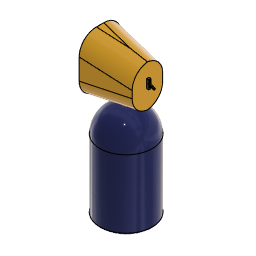
WeirdLamp v2 (Autodesk Fusion 360 design; units mm, degrees)
Autodesk Fusion 360 part; units mm, degrees
sketch "Sketch1" plane through (0, 0, 0) normal (0, 0, 1) x (1, 0, 0)
  circle A0 centre (0, 0) radius 37.5
  dimension "d1" = 75
  constraint coincident A0.centre origin
  measures "d1" diameter of A0
extrude "Extrude1" add sketch "Sketch1" along normal blind 100 makes body 1
sphere "SpherePrimitive1" add diameter 75 placed x (-1, 0, 0) y (0, -1, 0) z (0, 0, 1) at (0, 0, 100) separate body makes body 2
combine "Combine1" operation add target body 2 tool bodies 1
ref_plane "WorkPlane1" through (0, 0, 137.5) normal (0, 0, -1) x (-1, 0, 0)
sketch "Sketch3" plane through (0, 0, 137.5) normal (0, 0, -1) x (1, 0, 0)
  circle A0 centre (0, 0) radius 4.9069
  constraint coincident A0.centre origin
extrude "Extrude2" add sketch "Sketch3" along normal mid plane 78 separate body makes body 3
fillet "Fillet1" radius 2.5 1 edges at (-34.9623, -13.5606, 0) on bodies 2
ref_plane "WorkPlane2" through (-4.9069, 0, 176.5) normal (-1, 0, 0) x (0, -1, 0)
ref_plane "WorkPlane3" through (-37.5, 0, 98.5) normal (-1, 0, 0) x (0, -1, 0)
sketch "Sketch5" plane through (-37.5, 0, 98.5) normal (-1, 0, 0) x (0, 1, 0)
  line L0 (-30, -38.0519) -> (30, -38.0519)
  line L1 (30, -38.0519) -> (30, -118.0519)
  line L2 (30, -118.0519) -> (-30, -118.0519)
  line L3 (-30, -118.0519) -> (-30, -38.0519)
  dimension "d12" = 60
  dimension "d13" = 80
  constraint horizontal L0
  constraint vertical L1
  constraint horizontal L2
  constraint vertical L3
  measures "d12" distance of L0.start L0.end
  measures "d13" distance of L0.start L2.end
ref_plane "WorkPlane4" through (32.5, 0, 176.5519) normal (-1, 0, 0) x (0, 1, 0)
sketch "Sketch6" plane through (32.5, 0, 176.5519) normal (-1, 0, 0) x (0, 1, 0)
  line L0 (20, -30) -> (-23.8137, -30)
  line L1 (-23.8137, -30) -> (-23.8137, 30)
  line L2 (-23.8137, 30) -> (20, 30)
  line L3 (20, 30) -> (20, -30)
  dimension "d17" = 43.8137
  dimension "d18" = 60
  constraint horizontal L0
  constraint vertical L1
  constraint horizontal L2
  constraint vertical L3
  measures "d17" distance of L0.start L0.end
  measures "d18" distance of L0.start L2.end
loft "Loft1" add profiles "Sketch6", "Sketch5" section 1 section 2 separate body makes body 4
fillet "Fillet2" radius 25 4 edges at (-2.5, 25, 141.5519) (-2.5, 25, 211.5519) (-2.5, -26.9068, 211.5519) (-2.5, -26.9068, 141.5519) on bodies 4
hole "Hole1" at (-37.5, 0.0166, 176.5519) direction (1, 0, 0) diameter 30 depth 50 tip angle 118 bodies 3 4
hole "Hole2" at (-0.3526, 0.0166, 161.5519) direction (0, 0, -1) diameter 5 depth 69 tip angle 118 bodies 2 3
sketch "Sketch7" plane through (32.5, 0, 0) normal (1, 0, 0) x (0, 1, 0)
  ellipse E0 centre (1.2838, 171.8057) end of major axis (-12.053, 150.2473) minor radius 25 (-23.8137, 171.4913) -> (-1.8806, 146.7158) ccw
  ellipse E1 centre (-5.2538, 171.8057) end of major axis (12.781, 153.7709) minor radius 25 (-1.8806, 146.7158) -> (20, 171.3007) ccw
  line L0 (20, 171.3007) -> (20, 181.8032)
  ellipse E2 centre (-5.2538, 181.2981) end of major axis (12.781, 199.3329) minor radius 25 (20, 181.8032) -> (-1.8806, 206.3881) ccw
  ellipse E3 centre (1.2838, 181.2981) end of major axis (-12.053, 202.8566) minor radius 25 (-1.8806, 206.3881) -> (-23.8137, 181.6125) ccw
  line L1 (-23.8137, 181.6125) -> (-23.8137, 171.4913)
  line L2 (-3.0618, 186.2603) -> (0.1342, 186.2603)
  line L3 (0.1342, 186.2603) -> (0.1342, 173.6324)
  line L4 (0.1342, 173.6324) -> (-3.0618, 173.6324)
  line L5 (-3.0618, 173.6324) -> (-3.0618, 186.2603)
  constraint horizontal L2
  constraint vertical L3
  constraint horizontal L4
  constraint vertical L5
extrude "Extrude3" add sketch "Sketch7" along normal blind 3 separate body contours L2 L3 L4 L5 makes body 5
sketch "Sketch8" plane through (35.5, 0, 0) normal (1, 0, 0) x (0, 1, 0)
  line L0 (-3.0618, 173.6324) -> (0.1342, 173.6324)
  line L1 (0.1342, 173.6324) -> (0.1342, 186.2603)
  line L2 (0.1342, 186.2603) -> (-3.0618, 186.2603)
  line L3 (-3.0618, 186.2603) -> (-3.0618, 173.6324)
  line L4 (-2.2612, 185.1367) -> (-0.7022, 185.1367)
  line L5 (-0.7022, 185.1367) -> (-0.7022, 175.393)
  line L6 (-0.7022, 175.393) -> (-2.2612, 175.393)
  line L7 (-2.2612, 175.393) -> (-2.2612, 185.1367)
  constraint horizontal L4
  constraint vertical L5
  constraint horizontal L6
  constraint vertical L7
extrude "Extrude4" cut sketch "Sketch8" against normal blind 2 contours L4 L5 L6 L7 bodies 5
sketch "Sketch9" plane through (33.5, 0, 0) normal (1, 0, 0) x (0, 1, 0)
  line L0 (-2.2612, 175.393) -> (-0.7022, 175.393)
  line L1 (-0.7022, 175.393) -> (-0.7022, 185.1367)
  line L2 (-0.7022, 185.1367) -> (-2.2612, 185.1367)
  line L3 (-2.2612, 185.1367) -> (-2.2612, 175.393)
  line L4 (-2.2612, 181.8711) -> (-0.7022, 181.8711)
  line L5 (-0.7022, 181.8711) -> (-0.7022, 180.2648)
  line L6 (-0.7022, 180.2648) -> (-2.2612, 180.2648)
  line L7 (-2.2612, 180.2648) -> (-2.2612, 181.8711)
  constraint horizontal L4
  constraint vertical L5
  constraint horizontal L6
  constraint vertical L7
  constraint coincident L1 L5.end
  constraint coincident L3 L4.start
  constraint midpoint L1 L5.end
extrude "Extrude5" add sketch "Sketch9" along normal blind 9 separate body contours L1 L3 L4 L5 L6 L7 makes body 6
copy_body "Body->Comp1" bodies 6 removing the originals makes body 7 in component "Component"
copy_body "Body->Comp2" bodies 5 removing the originals makes body 8 in component "Component'"
component "Component" placed x (0.906308, 0, -0.422618) y (0.422618, 0, 0.906308) z (0, -1, 0) at (4.5943, 179.5061, 196.1534)
component "Component'" placed x (1, 0, 0) y (0, 1, 0) z (0, 0, 1) at (0, 0, 0)
